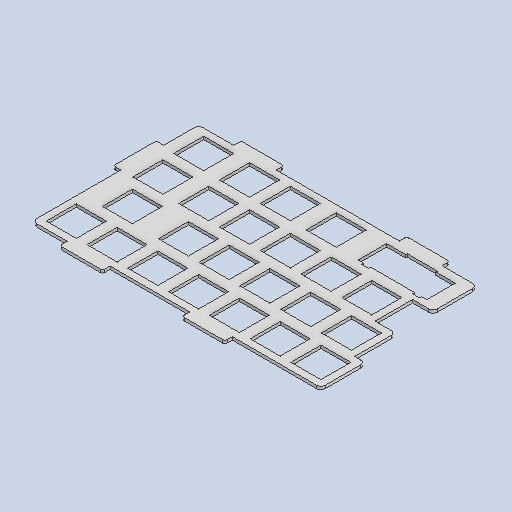
# Autodesk Inventor part: Plate_Right
Saved by Autodesk Inventor 2023 (Build 270158000, 158)
## iProperties
Created: 2022-11-13
Part Number: Plate_Right
Material: Generic
Document SubType Name: Modeling
Designer: reide
Density: 1 g/cm^3
Appearance: Default
Author: reide
Autodesk Inventor part; units mm, degrees
ref_plane "YZ Plane" through (0, 0, 0) normal (1, 0, 0) x (0, 1, 0)
ref_plane "XZ Plane" through (0, 0, 0) normal (0, 1, 0) x (-1, 0, 0)
ref_plane "XY Plane" through (0, 0, 0) normal (0, 0, 1) x (1, 0, 0)
sketch "Sketch1" plane through (0, 0, 0) normal (0, 1, 0) x (-1, 0, 0)
  line L0 (134.85, 0) -> (0, 0)
  line L1 (0, -20.55) -> (0, 0)
  line L2 (4.7625, -20.55) -> (0, -20.55)
  line L3 (4.7625, -39.6) -> (4.7625, -20.55)
  line L4 (14.2875, -39.6) -> (4.7625, -39.6)
  line L5 (14.2875, -57.15) -> (14.2875, -39.6)
  line L6 (4.7625, -57.15) -> (14.2875, -57.15)
  line L7 (4.7625, -77.7) -> (4.7625, -57.15)
  line L8 (4.7625, -77.7) -> (134.85, -77.7)
  line L9 (134.85, -77.7) -> (134.85, 0)
  line L10 (16.693, -60.425) -> (37.1941, -60.425)
  line L11 (37.1941, -60.425) -> (37.1941, -59.4549)
  line L12 (37.1941, -59.4549) -> (40.4931, -59.4549)
  line L13 (40.4931, -59.4549) -> (40.4931, -60.425)
  line L14 (40.4931, -60.425) -> (42.9684, -60.425)
  line L15 (42.9684, -60.425) -> (42.9684, -73.7043)
  line L16 (42.9684, -73.7043) -> (33.9433, -73.7043)
  line L17 (33.9433, -73.7043) -> (33.9433, -74.4243)
  line L18 (33.9433, -74.4243) -> (19.9438, -74.4243)
  line L19 (19.9438, -74.4243) -> (19.9438, -73.7043)
  line L20 (19.9438, -73.7043) -> (10.9188, -73.7043)
  line L21 (10.9188, -73.7043) -> (10.9188, -60.425)
  line L22 (10.9188, -60.425) -> (13.394, -60.425)
  line L23 (13.394, -60.425) -> (13.394, -59.4549)
  line L24 (13.394, -59.4549) -> (16.693, -59.4549)
  line L25 (16.693, -59.4549) -> (16.693, -60.425)
  line L26 (3.275, -17.275) -> (3.275, -3.275)
  line L27 (3.275, -3.275) -> (17.275, -3.275)
  line L28 (17.275, -3.275) -> (17.275, -17.275)
  line L29 (17.275, -17.275) -> (3.275, -17.275)
  line L30 (22.325, -17.275) -> (22.325, -3.275)
  line L31 (22.325, -3.275) -> (36.325, -3.275)
  line L32 (36.325, -3.275) -> (36.325, -17.275)
  line L33 (36.325, -17.275) -> (22.325, -17.275)
  line L34 (41.375, -17.275) -> (41.375, -3.275)
  line L35 (41.375, -3.275) -> (55.375, -3.275)
  line L36 (55.375, -3.275) -> (55.375, -17.275)
  line L37 (55.375, -17.275) -> (41.375, -17.275)
  line L38 (60.425, -17.275) -> (60.425, -3.275)
  line L39 (60.425, -3.275) -> (74.425, -3.275)
  line L40 (74.425, -3.275) -> (74.425, -17.275)
  line L41 (74.425, -17.275) -> (60.425, -17.275)
  line L42 (79.475, -17.275) -> (79.475, -3.275)
  line L43 (79.475, -3.275) -> (93.475, -3.275)
  line L44 (93.475, -3.275) -> (93.475, -17.275)
  line L45 (93.475, -17.275) -> (79.475, -17.275)
  line L46 (98.525, -17.275) -> (98.525, -3.275)
  line L47 (98.525, -3.275) -> (112.525, -3.275)
  line L48 (112.525, -3.275) -> (112.525, -17.275)
  line L49 (112.525, -17.275) -> (98.525, -17.275)
  line L50 (117.575, -17.275) -> (117.575, -3.275)
  line L51 (117.575, -3.275) -> (131.575, -3.275)
  line L52 (131.575, -3.275) -> (131.575, -17.275)
  line L53 (131.575, -17.275) -> (117.575, -17.275)
  line L54 (8.0375, -36.325) -> (8.0375, -22.325)
  line L55 (8.0375, -22.325) -> (22.0375, -22.325)
  line L56 (22.0375, -22.325) -> (22.0375, -36.325)
  line L57 (22.0375, -36.325) -> (8.0375, -36.325)
  line L58 (27.0875, -36.325) -> (27.0875, -22.325)
  line L59 (27.0875, -22.325) -> (41.0875, -22.325)
  line L60 (41.0875, -22.325) -> (41.0875, -36.325)
  line L61 (41.0875, -36.325) -> (27.0875, -36.325)
  line L62 (46.1375, -36.325) -> (46.1375, -22.325)
  line L63 (46.1375, -22.325) -> (60.1375, -22.325)
  line L64 (60.1375, -22.325) -> (60.1375, -36.325)
  line L65 (60.1375, -36.325) -> (46.1375, -36.325)
  line L66 (65.1875, -36.325) -> (65.1875, -22.325)
  line L67 (65.1875, -22.325) -> (79.1875, -22.325)
  line L68 (79.1875, -22.325) -> (79.1875, -36.325)
  line L69 (79.1875, -36.325) -> (65.1875, -36.325)
  line L70 (84.2375, -36.325) -> (84.2375, -22.325)
  line L71 (84.2375, -22.325) -> (98.2375, -22.325)
  line L72 (98.2375, -22.325) -> (98.2375, -36.325)
  line L73 (98.2375, -36.325) -> (84.2375, -36.325)
  line L74 (17.5625, -55.375) -> (17.5625, -41.375)
  line L75 (17.5625, -41.375) -> (31.5625, -41.375)
  line L76 (31.5625, -41.375) -> (31.5625, -55.375)
  line L77 (31.5625, -55.375) -> (17.5625, -55.375)
  line L78 (36.6125, -55.375) -> (36.6125, -41.375)
  line L79 (36.6125, -41.375) -> (50.6125, -41.375)
  line L80 (50.6125, -41.375) -> (50.6125, -55.375)
  line L81 (50.6125, -55.375) -> (36.6125, -55.375)
  line L82 (55.6625, -55.375) -> (55.6625, -41.375)
  line L83 (55.6625, -41.375) -> (69.6625, -41.375)
  line L84 (69.6625, -41.375) -> (69.6625, -55.375)
  line L85 (69.6625, -55.375) -> (55.6625, -55.375)
  line L86 (74.7125, -55.375) -> (74.7125, -41.375)
  line L87 (74.7125, -41.375) -> (88.7125, -41.375)
  line L88 (88.7125, -41.375) -> (88.7125, -55.375)
  line L89 (88.7125, -55.375) -> (74.7125, -55.375)
  line L90 (93.7625, -55.375) -> (93.7625, -41.375)
  line L91 (93.7625, -41.375) -> (107.7625, -41.375)
  line L92 (107.7625, -41.375) -> (107.7625, -55.375)
  line L93 (107.7625, -55.375) -> (93.7625, -55.375)
  line L94 (110.4312, -36.325) -> (110.4312, -22.325)
  line L95 (110.4312, -22.325) -> (124.4312, -22.325)
  line L96 (124.4312, -22.325) -> (124.4312, -36.325)
  line L97 (124.4312, -36.325) -> (110.4312, -36.325)
  line L98 (115.1937, -55.375) -> (115.1937, -41.375)
  line L99 (115.1937, -41.375) -> (129.1937, -41.375)
  line L100 (129.1937, -41.375) -> (129.1937, -55.375)
  line L101 (129.1937, -55.375) -> (115.1937, -55.375)
  line L102 (115.1937, -74.425) -> (115.1937, -60.425)
  line L103 (115.1937, -60.425) -> (129.1937, -60.425)
  line L104 (129.1937, -60.425) -> (129.1937, -74.425)
  line L105 (129.1937, -74.425) -> (115.1937, -74.425)
  line L106 (53.2813, -74.425) -> (53.2813, -60.425)
  line L107 (53.2813, -60.425) -> (67.2813, -60.425)
  line L108 (67.2813, -60.425) -> (67.2813, -74.425)
  line L109 (67.2813, -74.425) -> (53.2813, -74.425)
  line L110 (74.7125, -74.425) -> (74.7125, -60.425)
  line L111 (74.7125, -60.425) -> (88.7125, -60.425)
  line L112 (88.7125, -60.425) -> (88.7125, -74.425)
  line L113 (88.7125, -74.425) -> (74.7125, -74.425)
  line L114 (93.7625, -74.425) -> (93.7625, -60.425)
  line L115 (93.7625, -60.425) -> (107.7625, -60.425)
  line L116 (107.7625, -60.425) -> (107.7625, -74.425)
  line L117 (107.7625, -74.425) -> (93.7625, -74.425)
  line L118 (98.525, 0) -> (118.525, 0)
  line L119 (118.525, 0) -> (118.525, 3.5)
  line L120 (118.525, 3.5) -> (98.525, 3.5)
  line L121 (98.525, 3.5) -> (98.525, 0)
  arc A0 (12, -0.75) -> (16, 3.25) centre (12, 3.25) ccw projected
  line L122 (2.775, -0.75) -> (12, -0.75) projected
  line L123 (2.775, -18.775) -> (2.775, -0.75) projected
  arc A1 (7.5375, -24.646) -> (2.775, -18.775) centre (1.5375, -24.646) ccw projected
  line L124 (7.5375, -37.825) -> (7.5375, -24.646) projected
  line L125 (11.0625, -37.825) -> (7.5375, -37.825) projected
  arc A2 (17.0625, -43.825) -> (11.0625, -37.825) centre (11.0625, -43.825) ccw projected
  line L126 (17.0625, -49.375) -> (17.0625, -43.825) projected
  arc A3 (11.0625, -55.375) -> (17.0625, -49.375) centre (11.0625, -49.375) ccw projected
  line L127 (11.0625, -55.375) -> (7.5375, -55.375) projected
  line L128 (7.5375, -76.95) -> (7.5375, -55.375) projected
  line L129 (11.6688, -76.95) -> (7.5375, -76.95) projected
  line L130 (11.6688, -77.95) -> (11.6688, -76.95) projected
  line L131 (11.6688, -77.95) -> (42.2184, -77.95) projected
  line L132 (42.2184, -76.95) -> (42.2184, -77.95) projected
  line L133 (133.6, -76.95) -> (42.2184, -76.95) projected
  line L134 (133.6, -76.95) -> (133.6, -40.364) projected
  line L135 (133.6, -40.364) -> (135.1, -40.364) projected
  line L136 (135.1, -40.364) -> (135.1, -34.864) projected
  line L137 (135.1, -34.864) -> (136.1, -34.864) projected
  line L138 (136.1, -34.864) -> (136.1, -36.864) projected
  line L139 (136.1, -36.864) -> (140.1, -36.864) projected
  line L140 (140.1, -36.864) -> (140.1, -79.95) projected
  arc A4 (137.1, -82.95) -> (140.1, -79.95) centre (137.1, -79.95) ccw projected
  line L141 (137.1, -82.95) -> (-3.25, -82.95) projected
  line L142 (-3.25, -82.95) -> (-3.25, 6.75) projected
  line L143 (-3.25, 6.75) -> (16, 6.75) projected
  line L144 (16, 3.25) -> (16, 6.75) projected
  circle A5 centre (68.425, -79.45) radius 1.5 projected
  circle A6 centre (136.6, -47.95) radius 1.5 projected
  circle A7 centre (1, -37.95) radius 1.5 projected
  circle A8 centre (1, -78.7) radius 1.5 projected
  circle A9 centre (1, 2.5) radius 1.5 projected
  circle A10 centre (136.6, -79.45) radius 1.5 projected
  arc A11 (34, 3.25) -> (38, -0.75) centre (38, 3.25) ccw projected
  line L145 (34, 5.75) -> (34, 3.25) projected
  line L146 (30, 5.75) -> (34, 5.75) projected
  line L147 (30, 6.75) -> (30, 5.75) projected
  line L148 (30, 6.75) -> (137.1, 6.75) projected
  arc A12 (140.1, 3.75) -> (137.1, 6.75) centre (137.1, 3.75) ccw projected
  line L149 (140.1, 3.75) -> (140.1, -23.864) projected
  line L150 (140.1, -23.864) -> (136.1, -23.864) projected
  line L151 (136.1, -23.864) -> (136.1, -25.864) projected
  line L152 (136.1, -25.864) -> (135.1, -25.864) projected
  line L153 (135.1, -25.864) -> (135.1, -20.364) projected
  line L154 (135.1, -20.364) -> (133.6, -20.364) projected
  line L155 (133.6, -20.364) -> (133.6, -0.75) projected
  line L156 (38, -0.75) -> (133.6, -0.75) projected
  circle A13 centre (135.85, 2.5) radius 1.5 projected
  circle A14 centre (68.425, 2.5) radius 1.5 projected
  line L157 (41.375, 0) -> (61.375, 0)
  line L158 (61.375, 0) -> (61.375, 3.5)
  line L159 (61.375, 3.5) -> (41.375, 3.5)
  line L160 (41.375, 3.5) -> (41.375, 0)
  line L161 (98.525, -77.7) -> (118.525, -77.7)
  line L162 (118.525, -77.7) -> (118.525, -81.2)
  line L163 (118.525, -81.2) -> (98.525, -81.2)
  line L164 (98.525, -81.2) -> (98.525, -77.7)
  line L165 (69.8062, -77.7) -> (69.8062, -87)
  line L166 (134.85, -77.7) -> (4.7625, -77.7)
  line L167 (41.0875, -77.7) -> (21.0875, -77.7)
  line L168 (21.0875, -77.7) -> (21.0875, -81.2)
  line L169 (21.0875, -81.2) -> (41.0875, -81.2)
  line L170 (41.0875, -81.2) -> (41.0875, -77.7)
  line L171 (134.85, -41.375) -> (134.85, -61.375)
  line L172 (134.85, -61.375) -> (138.35, -61.375)
  line L173 (138.35, -61.375) -> (138.35, -41.375)
  line L174 (138.35, -41.375) -> (134.85, -41.375)
  point P0 (0.75, -0.75)
  dimension "d3" = 20
  dimension "d4" = 3.5
  dimension "d5" = 20
  dimension "d6" = 3.5
  dimension "d7" = 3.5
  dimension "d8" = 20
  dimension "d9" = 3.5
  constraints: 280 end point, 11 perpendicular, 10 point on line, 6 symmetric about line, 1 midpoint, 1 parallel, 1 vertical
  measures "d3" distance of L118.start L118.end
  measures "d4" distance of L118.end L119.end
  measures "d5" distance of L157.start L157.end
  measures "d6" distance of L157.end L158.end
  measures "d7" distance of L161.end L162.end
  measures "d8" distance of L171.start L171.end
  measures "d9" distance of L171.end L172.end
extrude "Extrusion1" add sketch "Sketch1" along normal blind 1.4 contours L9 L154 L155 L156 A11 L0 | L0 L121 L120 L119 | L9 L135 L134 L133 L132 L8 L130 L129 L128 L6 L5 A3 L126 A2 L125 L124 A1 L123 L122 A0 L0 A11 L156 L155 L154 | L9 L8 L132 L133 L134 L135 | L0 L160 L159 L158 | L174 L173 L172 L9 | A0 L122 L123 A1 L124 L125 A2 L126 A3 L5 L4 L3 L2 L1 L0 | L162 L163 L164 L8 | L170 L131 L168 L8 | L170 L169 L168 L131 | L8 L7 L6 L128 L129 L130 | A6
fillet "Fillet1" radius 2 7 edges at (-134.85, 0.7, -77.7) (-4.7625, 0.7, -77.7) (0, 0.7, 0) (-134.85, 0.7, 0) (0, 0.7, -20.55) (-4.7625, 0.7, -39.6) (-4.7625, 0.7, -57.15)
fillet "Fillet2" radius 1 10 edges at (-21.0875, 0.7, -81.2) (-41.0875, 0.7, -81.2) (-98.525, 0.7, -81.2) (-118.525, 0.7, -81.2) (-138.35, 0.7, -61.375) (-138.35, 0.7, -41.375) (-118.525, 0.7, 3.5) (-98.525, 0.7, 3.5) (-41.375, 0.7, 3.5) (-61.375, 0.7, 3.5)
body "Solid1"
